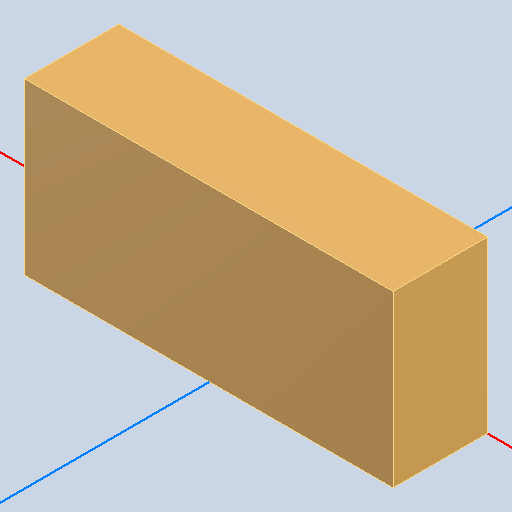
# Autodesk Inventor part: CGRM4004-G
Saved by Autodesk Inventor 2022 (Build 260153000, 153)
## iProperties
Created: 2022-12-24
Part Number: CGRM4004-G
Material: Типовые
Document SubType Name: Modeling
Designer: Ivan Petrov
Density: 1 g/cm^3
Appearance: SOD-123_MINI-SMA, CGRM4004-G
Author: Ivan Petrov
Autodesk Inventor part; units mm, degrees
ref_plane "YZ Plane" through (0, 0, 0) normal (1, 0, 0) x (0, 1, 0)
ref_plane "XZ Plane" through (0, 0, 0) normal (0, 1, 0) x (-1, 0, 0)
ref_plane "XY Plane" through (0, 0, 0) normal (0, 0, 1) x (1, 0, 0)
sketch "SOD-123_MINI-SMA, CGRM4004-G_13" plane through (0, 0, 0) normal (0, 0, 1) x (1, 0, 0)
  line L0 (-1.95, 0.9) -> (1.95, 0.9)
  line L1 (1.95, 0.9) -> (1.95, -0.9)
  line L2 (1.95, -0.9) -> (-1.95, -0.9)
  line L3 (-1.95, -0.9) -> (-1.95, 0.9)
  constraints: 8 end point
extrude "Выдавливание1" add sketch "SOD-123_MINI-SMA, CGRM4004-G_13" along normal blind 1
